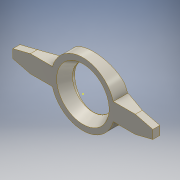
# Autodesk Inventor part: HeadBar
Saved by Autodesk Inventor 2016 (Build 200138000, 138)
## iProperties
Created: 2015-11-18
Part Number: HeadBar
Material: Titanium
Document SubType Name: Modeling
Designer: Vervaeke-Lab
Density: 4.51 g/cm^3
Appearance: Titanium
Mass: 0.799757 g
Surface Area: 3.59174 cm^2
Volume: 0.17733 cm^3
Author: Vervaeke-Lab
Autodesk Inventor part; units mm, degrees
ref_plane "YZ Plane" through (0, 0, 0) normal (1, 0, 0) x (0, 1, 0)
ref_plane "XZ Plane" through (0, 0, 0) normal (0, 1, 0) x (-1, 0, 0)
ref_plane "XY Plane" through (0, 0, 0) normal (0, 0, 1) x (1, 0, 0)
sketch "Sketch1" plane through (0, 0, 0) normal (0, 1, 0) x (-1, 0, 0)
  circle A0 centre (0, 0) radius 4.8
  line L0 (5.5749, -1.6) -> (9.6, -1.6)
  line L1 (9.6, -1.6) -> (12.8, -0.8)
  line L2 (12.8, -0.8) -> (12.8, 0.8)
  line L3 (12.8, 0.8) -> (9.6, 1.6)
  line L4 (9.6, 1.6) -> (5.5749, 1.6)
  arc A1 (5.5749, 1.6) -> (-5.5704, 1.6) centre (0.0023, -0.0079) ccw
  line L5 (-5.5704, 1.6) -> (-9.6, 1.6)
  line L6 (-5.5704, -1.6) -> (-9.5955, -1.6)
  line L7 (-9.5955, -1.6) -> (-12.7955, -0.8)
  line L8 (-12.7955, -0.8) -> (-12.7955, 0.8)
  line L9 (-12.7955, 0.8) -> (-9.5955, 1.6)
  line L10 (-9.5955, 1.6) -> (-5.5704, 1.6)
  arc A2 (-5.5704, -1.6) -> (5.5749, -1.6) centre (0.0023, -0.0158) ccw
  circle A3 centre (0.0023, -0.0158) radius 3.8
  point P0 (-9.6, -1.207)
  dimension "d0" = 9.6
  dimension "d9" = 7.6
  constraints: 22 end point, 4 centre point, 4 point on circle, 2 coincident, 2 horizontal, 1 parallel, 1 perpendicular, 1 point on line
  measures "d0" diameter of A0
  measures "d9" diameter of A3
extrude "Extrusion1" add sketch "Sketch1" along normal blind 2.6 contours A0 | A2 L6 L7 L8 L9 L5 A1 L4 L3 L2 L1 L0
sketch "Sketch16" plane through (0, 0, 0) normal (0, 0, 1) x (1, 0, 0)
  line L0 (12.7955, 0) -> (12.7955, 2.6) projected
  line L1 (12.7955, 1.27) -> (9.5955, 1.27)
  line L2 (9.5955, 0) -> (9.5955, 2.6) projected
  line L3 (9.5955, 1.27) -> (5.8, 2.6)
  arc A0 (-5, 2.6) -> (5, 2.6) centre (0, 20.1101) ccw
  line L4 (-9.6, 0) -> (-9.6, 2.6) projected
  line L5 (12.7955, 1.27) -> (12.7955, 5.6941)
  line L6 (-12.8, 0) -> (-12.8, 2.6) projected
  line L7 (-12.8, 1.27) -> (-12.8, 6.6119)
  line L8 (-12.8, 6.6119) -> (12.7955, 5.6941)
  line L9 (5.8, 2.6) -> (5, 2.6)
  line L10 (-5, 2.6) -> (-5.8, 2.6)
  line L11 (-5.8, 2.6) -> (-9.6, 1.27)
  line L12 (-9.6, 1.27) -> (-12.8, 1.27)
  line L13 (9.5955, 1.27) -> (5.8, 2.6)
  line L14 (9.5955, 1.27) -> (5.8, 2.6)
  line L15 (5.8, 2.6) -> (5, 2.6)
  point P0 (0, 0)
  dimension "d5" = 10
  dimension "d6" = 18.21
  constraints: 24 end point, 4 point on line, 3 coincident, 3 collinear, 2 horizontal, 2 point on circle, 1 centre point, 1 perpendicular, 1 vertical
  measures "d5" distance of L9.end L10.start
  measures "d6" radius of A0
extrude "Extrusion3" cut sketch "Sketch16" along normal mid plane 12
sketch "Sketch17" plane through (0, 0, 0) normal (0, 0, 1) x (1, 0, 0)
  point P0 (0, 0)
sketch "Sketch18" plane through (0, 0, 0) normal (0, 0, 1) x (1, 0, 0)
  line L0 (-3.8023, 0) -> (-3.8023, 2.3015) projected
  line L1 (-3.8023, 1.8964) -> (0, 1.8964)
  line L2 (3.7977, 0) -> (3.7977, 2.3005) projected
  line L3 (-5.5749, 0) -> (5.5704, 0) projected
  line L4 (3.7977, 1.8964) -> (5.9415, 1.8964) construction
  line L5 (-3.8023, 1.8964) -> (-4.8021, 0)
  line L6 (-3.8023, 1.8964) -> (-1.6585, 1.8964) construction
  line L7 (0, 0) -> (0, 1.9)
  line L8 (0, 0) -> (-4.8021, 0)
  dimension "d11" = 117.8
  constraints: 13 end point, 3 horizontal, 3 point on line, 1 collinear, 1 equal length, 1 vertical
  measures "d11" angle of L5 L6
revolve "Revolution1" cut sketch "Sketch18" angle 360 about axis through (0, 0, 0) along (0, 1, 0)
body "Solid1"
